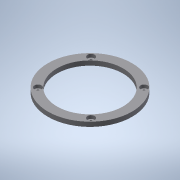
# Autodesk Inventor part: chamberPlateCircle
Saved by Autodesk Inventor 2021 (Build 250183000, 183)
## iProperties
Created: 2016-06-27
Part Number: chamberPlateCircle
Material: Generic
Document SubType Name: Modeling
Designer: 120pa
Density: 1 g/cm^3
Appearance: Default
Author: 120pa
Autodesk Inventor part; units mm, degrees
ref_plane "YZ Plane" through (0, 0, 0) normal (1, 0, 0) x (0, 1, 0)
ref_plane "XZ Plane" through (0, 0, 0) normal (0, 1, 0) x (-1, 0, 0)
ref_plane "XY Plane" through (0, 0, 0) normal (0, 0, 1) x (1, 0, 0)
sketch "Sketch1" plane through (0, 0, 0) normal (0, 1, 0) x (-1, 0, 0)
  circle A0 centre (0, 0) radius 22
  circle A1 centre (0, 0) radius 28
  dimension "d0" = 44
  dimension "d1" = 56
  constraints: 2 centre point
  measures "d0" diameter of A0
  measures "d1" diameter of A1
extrude "Extrusion1" add sketch "Sketch1" along normal blind 3
sketch "Sketch5" plane through (0, 3, 0) normal (0, 1, 0) x (1, 0, 0)
  line L0 (18.0303, 18.03) -> (-17.325, 18.03)
  line L1 (-17.325, 18.03) -> (-17.325, -17.325)
  line L2 (-17.325, -17.325) -> (18.0303, -17.325)
  line L3 (18.0303, -17.325) -> (18.0303, 18.03)
  point P0 (0, 0)
  dimension "d22" = 35.3553
  dimension "d23" = 35.355
  constraints: 8 end point, 2 parallel, 1 horizontal, 1 perpendicular
  measures "d22" distance of L2.end L1.end
  measures "d23" distance of L1.end L0.end
hole "Hole3" at (-17.325, 3, 17.325) at (-17.325, 3, -18.03) at (18.0303, 3, -18.03) at (18.0303, 3, 17.325) direction (0, -1, 0) diameter 2.438 end through all counterbore diameter 4.763 counterbore depth 2.184 clearance for "Socket Head Cap Screw" size "#2" standard "Ansi Unified Screw Threads"
body "Solid1"
